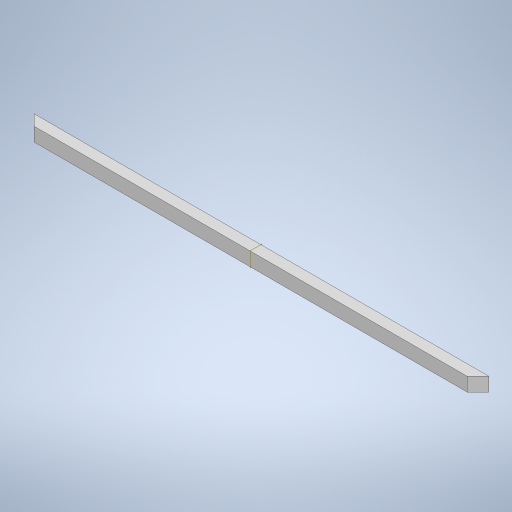
# Autodesk Inventor part: lengthBinding
Saved by Autodesk Inventor 2024.2 (Build 282272000, 272)
## iProperties
Created: 2024-06-09
Part Number: lengthBinding
Material: Generic
Document SubType Name: Modeling
Designer: user
Density: 1 g/cm^3
Appearance: Default
Author: user
Autodesk Inventor part; units mm, degrees
ref_plane "YZ Plane" through (0, 0, 0) normal (1, 0, 0) x (0, 1, 0)
ref_plane "XZ Plane" through (0, 0, 0) normal (0, 1, 0) x (-1, 0, 0)
ref_plane "XY Plane" through (0, 0, 0) normal (0, 0, 1) x (1, 0, 0)
sketch "Sketch1" plane through (0, 0, 0) normal (0, 0, 1) x (1, 0, 0)
  line L0 (315, -9.5) -> (-315, -9.5)
  line L1 (-315, -9.5) -> (-315, 9.5)
  line L2 (-315, 9.5) -> (315, 9.5)
  line L3 (315, 9.5) -> (315, -9.5)
  line L4 (315, -9.5) -> (-315, 9.5) construction
  line L5 (-315, -9.5) -> (315, 9.5) construction
  point P0 (0, 0)
  dimension "d0" = 630
  dimension "d1" = 19
  constraints: 12 end point, 2 midpoint, 2 parallel, 1 horizontal, 1 perpendicular
  measures "d0" distance of L1.end L2.end
  measures "d1" distance of L0.end L1.end
extrude "Extrusion1" add sketch "Sketch1" along normal blind 15
sketch "Sketch2" plane through (-315, 9.5, 0) normal (0, 1, 0) x (1, 0, 0)
  line L0 (630, 0) -> (0, 0) projected
  line L1 (0, 0) -> (15, -15)
  line L2 (630, -15) -> (0, -15) projected
  line L3 (15, -15) -> (0, -15)
  line L4 (0, -15) -> (0, 0)
  point P0 (315, 0)
  dimension "d4" = 45
  constraints: 6 end point, 1 collinear, 1 perpendicular, 1 point on line
  measures "d4" angle of L2 L1
extrude "Extrusion2" cut sketch "Sketch2" against normal through all
mirror "Mirror1" about plane through (0, 0, 0) normal (1, 0, 0) of "Extrusion2"
ref_plane "Work Plane1" through (0, 0, 0) normal (1, 0, 0) x (0, 1, 0)
body "Solid1"
